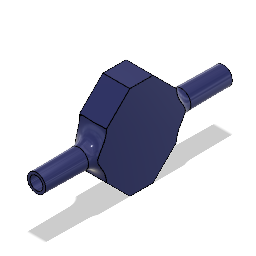
Sensor_Adapter (Autodesk Fusion 360 design; units mm, degrees)
Autodesk Fusion 360 part; units mm, degrees
sketch "Sketch1" plane through (0, 0, 0) normal (0, 0, 1) x (1, 0, 0)
  circle A0 centre (0, 0) radius 1.985
  dimension "d1" = 3.97
  measures "d1" diameter of A0
ref_plane "WorkPlane1" through (0, 0, 20) normal (0, 0, 1) x (1, 0, 0)
ref_plane "WorkPlane2" through (0, 0, 40) normal (0, 0, 1) x (1, 0, 0)
sketch "Sketch2" plane through (0, 0, 40) normal (0, 0, 1) x (1, 0, 0)
  circle A0 centre (0, 0) radius 1.985
  dimension "d7" = 3.97
  measures "d7" diameter of A0
ref_plane "WorkPlane3" through (0, 0, 27.5) normal (0, 0, 1) x (1, 0, 0)
ref_plane "WorkPlane4" through (0, 0, 12.5) normal (0, 0, 1) x (1, 0, 0)
sketch "Sketch3" plane through (0, 0, 27.5) normal (0, 0, 1) x (1, 0, 0)
  circle A0 centre (0, 0) radius 2.15
  dimension "d11" = 4.3
  measures "d11" diameter of A0
sketch "Sketch4" plane through (0, 0, 12.5) normal (0, 0, 1) x (1, 0, 0)
  circle A0 centre (0, 0) radius 2.15
  dimension "d13" = 4.3
  measures "d13" diameter of A0
loft "Loft1" add profiles "Sketch2", "Sketch3" section 1 section 2 makes body 1
loft "Loft2" add profiles "Sketch1", "Sketch4" section 1 section 2 separate body makes body 2
sketch "Sketch6" plane through (0, 0, 40) normal (0, 0, 1) x (1, 0, 0)
  circle A0 centre (0, 0) radius 1.985
  circle A1 centre (0, 0) radius 1.4
  dimension "d16" = 2.8
  measures "d16" diameter of A1
sketch "Sketch7" plane through (0, 0, 0) normal (0, 0, -1) x (-1, 0, 0)
  circle A0 centre (0, 0) radius 1.985
  circle A1 centre (0, 0) radius 1.4
  dimension "d17" = 2.8
  measures "d17" diameter of A1
extrude "Extrude1" cut sketch "Sketch6" against normal blind 10 contours A1 bodies 1
extrude "Extrude2" cut sketch "Sketch7" against normal blind 10 contours A1 bodies 2
sketch "Sketch8" plane through (0, 0, 20) normal (0, 0, 1) x (1, 0, 0)
  line L0 (2.5, -10) -> (-2.5, -10)
  line L1 (-2.5, -10) -> (-2.5, 10)
  line L2 (-2.5, 10) -> (2.5, 10)
  line L3 (2.5, 10) -> (2.5, -10)
  line L4 (2.5, -10) -> (-2.5, 10) construction
  line L5 (-2.5, -10) -> (2.5, 10) construction
  dimension "d22" = 5
  dimension "d23" = 20
extrude "Extrude3" add sketch "Sketch8" along normal mid plane 15 separate body makes body 3
combine "Combine1" operation add target body 2 tool bodies 3 1
extrude "Extrude8" cut 1 faces at (0.5498, -0.3174, 30) along direction (0, 0, -1) blind 20 on bodies 2 bodies 2
sketch "Sketch11" plane through (-2.5, 0, 0) normal (-1, 0, 0) x (0, 0, 1)
  line L0 (27.5, -10) -> (27.5, 10)
  line L1 (27.5, 10) -> (12.5, 10)
  line L2 (12.5, 10) -> (12.5, -10)
  line L3 (12.5, -10) -> (27.5, -10)
  circle A0 centre (20, 0) radius 2.9
  dimension "d42" = 5.8
  measures "d42" diameter of A0
extrude "Extrude9" cut sketch "Sketch11" against normal blind 3.6 contours A0 bodies 2
extrude "Extrude10" add 1 faces at (-2.5, 7.6306, 20.0722) along direction (-1, 0, 0) blind 0.8 on bodies 2 bodies 2
sketch "Sketch12" plane through (-3.3, 0, 0) normal (-1, 0, 0) x (0, 0, 1)
  circle A0 centre (20, 0) radius 2.9
  line L0 (12.5, -10) -> (27.5, -10)
  line L1 (27.5, -10) -> (27.5, 10)
  line L2 (27.5, 10) -> (12.5, 10)
  line L3 (12.5, 10) -> (12.5, -10)
  circle A1 centre (20, 7) radius 1.5
  circle A2 centre (20, -7) radius 1.5
  dimension "d48" = 3
  dimension "d49" = 7
  dimension "d50" = 3
  dimension "d51" = 7
  measures "d48" diameter of A1
  measures "d50" diameter of A2
extrude "Extrude11" cut sketch "Sketch12" against normal blind 2.9 contours A1 | A2 bodies 2
chamfer "Chamfer1" distance 5 angle 45 4 edges at (-0.4, 10, 27.5) (-0.4, 10, 12.5) (-0.4, -10, 12.5) (-0.4, -10, 27.5) on bodies 2
fillet "Fillet3" radius 3.5 2 edges at (-2.0045, 0.7775, 27.5) (-2.0045, 0.7775, 12.5) on bodies 2
equation "d1 = diameter_adapter"
equation "d2 = length_entrance_to_center"
equation "diameter_tubbing1 = 4 mm"
equation "diameter_adapter = 3.97 mm"
equation "length_entrance_to_center = 20 mm"
equation "d6 = length_entrance_to_center"
equation "d7 = diameter_adapter"
equation "length_tubbing_coverage = 12.5 mm"
equation "d9 = -length_tubbing_coverage"
equation "d10 = length_tubbing_coverage"
equation "d11 = diameter_tubbing2"
equation "diameter_tubbing2 = 4.3 mm"
equation "d13 = diameter_tubbing2"
equation "diameter_tubbing_inside = 2.8 mm"
equation "d16 = diameter_tubbing_inside"
equation "d17 = diameter_tubbing_inside"
equation "diameter_pressure_sensor = 5.8 mm"
equation "diameter_threaded_insert = 3 mm"
equation "d48 = diameter_threaded_insert"
equation "d50 = diameter_threaded_insert"
equation "d51 = d49"
